Autodesk Fusion 360 part; units mm, degrees
note: some values were not read from the file. Set by a fixed rule: which sketch regions a step uses.
(part 7 of 8)
  spline S678 degree 3 poles (31.6566, -63.6923) (31.72, -63.6389) (31.7978, -63.6072) (31.8772, -63.5903) knots 0 0 0 0 1 1 1 1
  spline S679 degree 3 poles (31.8772, -63.5903) (31.9567, -63.5733) (32.0382, -63.5705) (32.1192, -63.568) knots 0 0 0 0 1 1 1 1
  line L146 (32.1192, -63.568) -> (36.4524, -63.4348)
  spline S680 degree 3 poles (36.4524, -63.4348) (36.4673, -62.5804) (36.8861, -61.7442) (37.5474, -61.2485) knots 0 0 0 0 1 1 1 1
  spline S681 degree 3 poles (37.5474, -61.2485) (37.8359, -61.0322) (38.1674, -60.8807) (38.5136, -60.8015) knots 0 0 0 0 1 1 1 1
  spline S682 degree 3 poles (38.5136, -60.8015) (38.8597, -60.7222) (39.217, -60.719) (39.5712, -60.7246) knots 0 0 0 0 1 1 1 1
  line L147 (39.5712, -60.7246) -> (51.3095, -60.9089)
  spline S683 degree 3 poles (51.3095, -60.9089) (51.8749, -60.9209) (52.434, -61.1493) (52.859, -61.542) knots 0 0 0 0 1 1 1 1
  spline S684 degree 3 poles (52.859, -61.542) (53.2166, -61.8724) (53.4741, -62.3063) (53.6869, -62.7542) knots 0 0 0 0 1 1 1 1
  spline S685 degree 3 poles (53.6869, -62.7542) (53.7992, -62.9906) (53.9007, -63.2329) (54.0258, -63.462) knots 0 0 0 0 1 1 1 1
  spline S686 degree 3 poles (54.0258, -63.462) (54.151, -63.691) (54.3018, -63.9085) (54.4972, -64.0744) knots 0 0 0 0 1 1 1 1
  spline S687 degree 3 poles (54.4972, -64.0744) (54.8359, -64.3623) (55.2785, -64.4726) (55.7089, -64.5418) knots 0 0 0 0 1 1 1 1
  spline S688 degree 3 poles (55.7089, -64.5418) (56.3802, -64.6497) (57.0608, -64.6746) (57.7397, -64.6945) knots 0 0 0 0 1 1 1 1
  line L148 (57.7397, -64.6945) -> (115.1827, -66.374)
  spline S689 degree 3 poles (115.1827, -66.374) (115.5699, -66.3854) (115.96, -66.4334) (116.3432, -66.374) knots 0 0 0 0 1 1 1 1
  spline S690 degree 3 poles (116.3432, -66.374) (116.6033, -66.3338) (116.8559, -66.2316) (117.0685, -66.0687) knots 0 0 0 0 1 1 1 1
  spline S691 degree 3 poles (117.0685, -66.0687) (117.4625, -65.7668) (117.6901, -65.2882) (117.9389, -64.8472) knots 0 0 0 0 1 1 1 1
  spline S692 degree 3 poles (117.9389, -64.8472) (118.221, -64.3467) (118.5582, -63.8627) (119.0216, -63.5455) knots 0 0 0 0 1 1 1 1
  spline S693 degree 3 poles (119.0216, -63.5455) (119.4371, -63.2611) (119.943, -63.126) (120.437, -63.1676) knots 0 0 0 0 1 1 1 1
  line L149 (120.437, -63.1676) -> (132.5399, -63.4822)
  spline S694 degree 3 poles (132.5399, -63.4822) (133.197, -63.4272) (133.8722, -63.6945) (134.3319, -64.1917) knots 0 0 0 0 1 1 1 1
  spline S695 degree 3 poles (134.3319, -64.1917) (134.8295, -64.7298) (135.0609, -65.5271) (134.934, -66.2661) knots 0 0 0 0 1 1 1 1
  line L150 (134.934, -66.2661) -> (139.3401, -66.482)
  spline S696 degree 3 poles (139.3401, -66.482) (139.4661, -66.4882) (139.593, -66.4946) (139.7157, -66.5251) knots 0 0 0 0 1 1 1 1
  spline S697 degree 3 poles (139.7157, -66.5251) (139.8385, -66.5557) (139.9582, -66.6121) (140.0478, -66.7056) knots 0 0 0 0 1 1 1 1
  spline S698 degree 3 poles (140.0478, -66.7056) (140.1454, -66.8077) (140.2011, -66.9477) (140.2275, -67.0899) knots 0 0 0 0 1 1 1 1
  spline S699 degree 3 poles (140.2275, -67.0899) (140.254, -67.2321) (140.2535, -67.3781) (140.2528, -67.5231) knots 0 0 0 0 1 1 1 1
  line L151 (140.2528, -67.5231) -> (140.2444, -69.6792)
  spline S700 degree 3 poles (140.2444, -69.6792) (140.2439, -69.7923) (140.2433, -69.906) (140.2607, -70.0175) knots 0 0 0 0 1 1 1 1
  spline S701 degree 3 poles (140.2607, -70.0175) (140.2782, -70.129) (140.3152, -70.2397) (140.3843, -70.3262) knots 0 0 0 0 1 1 1 1
  spline S702 degree 3 poles (140.3843, -70.3262) (140.4319, -70.3858) (140.4939, -70.4324) (140.5628, -70.4604) knots 0 0 0 0 1 1 1 1
  spline S703 degree 3 poles (140.5628, -70.4604) (140.6318, -70.4884) (140.7074, -70.4978) (140.7806, -70.4874) knots 0 0 0 0 1 1 1 1
  line L152 (140.7806, -70.4874) -> (144.4775, -70.5414)
  spline S704 degree 3 poles (144.4775, -70.5414) (144.6381, -70.5658) (144.8078, -70.5118) (144.9287, -70.398) knots 0 0 0 0 1 1 1 1
  spline S705 degree 3 poles (144.9287, -70.398) (145.0669, -70.2678) (145.1365, -70.0617) (145.1075, -69.869) knots 0 0 0 0 1 1 1 1
  line L153 (145.1075, -69.869) -> (145.2012, -67.102)
  spline S706 degree 3 poles (145.2012, -67.102) (145.388, -66.9765) (145.5898, -66.8756) (145.8003, -66.8025) knots 0 0 0 0 1 1 1 1
  spline S707 degree 3 poles (145.8003, -66.8025) (146.3846, -66.5995) (147.0308, -66.6173) (147.6149, -66.8209) knots 0 0 0 0 1 1 1 1
  spline S708 degree 3 poles (147.6149, -66.8209) (148.199, -67.0245) (148.7207, -67.4089) (149.1271, -67.8952) knots 0 0 0 0 1 1 1 1
  spline S709 degree 3 poles (149.1271, -67.8952) (149.9398, -68.8679) (150.2708, -70.2083) (150.2564, -71.5036) knots 0 0 0 0 1 1 1 1
  spline S710 degree 3 poles (150.2564, -71.5036) (150.2364, -73.3042) (149.5784, -75.0893) (148.4395, -76.433) knots 0 0 0 0 1 1 1 1
  line L154 (148.4395, -76.433) -> (134.4244, -76.4161)
  spline S711 degree 3 poles (134.4244, -76.4161) (134.2986, -76.8823) (133.9928, -77.2916) (133.5922, -77.5304) knots 0 0 0 0 1 1 1 1
  spline S712 degree 3 poles (133.5922, -77.5304) (133.3009, -77.704) (132.9679, -77.7878) (132.6349, -77.8227) knots 0 0 0 0 1 1 1 1
  spline S713 degree 3 poles (132.6349, -77.8227) (132.3018, -77.8576) (131.9661, -77.846) (131.6316, -77.835) knots 0 0 0 0 1 1 1 1
  line L155 (131.6316, -77.835) -> (116.301, -77.3322)
  spline S714 degree 3 poles (116.301, -77.3322) (116.0942, -77.3254) (115.8862, -77.3195) (115.6817, -77.352) knots 0 0 0 0 1 1 1 1
  spline S715 degree 3 poles (115.6817, -77.352) (115.4771, -77.3844) (115.275, -77.4566) (115.1097, -77.5874) knots 0 0 0 0 1 1 1 1
  spline S716 degree 3 poles (115.1097, -77.5874) (114.9652, -77.7018) (114.8519, -77.8595) (114.7868, -78.0371) knots 0 0 0 0 1 1 1 1
  spline S717 degree 3 poles (114.7868, -78.0371) (114.7217, -78.2146) (114.7049, -78.4115) (114.7391, -78.5984) knots 0 0 0 0 1 1 1 1
  line L156 (114.7391, -78.5984) -> (114.679, -87.6426)
  spline S718 degree 3 poles (114.679, -87.6426) (114.6256, -88.1512) (114.8192, -88.6818) (115.1823, -89.0222) knots 0 0 0 0 1 1 1 1
  spline S719 degree 3 poles (115.1823, -89.0222) (115.4591, -89.2817) (115.8278, -89.4297) (116.1985, -89.4301) knots 0 0 0 0 1 1 1 1
  line L157 (116.1985, -89.4301) -> (132.3849, -90.0671)
  spline S720 degree 3 poles (132.3849, -90.0671) (132.8554, -90.0523) (133.3293, -90.2173) (133.6985, -90.5247) knots 0 0 0 0 1 1 1 1
  spline S721 degree 3 poles (133.6985, -90.5247) (134.111, -90.8681) (134.3875, -91.3869) (134.4509, -91.9364) knots 0 0 0 0 1 1 1 1
  line L158 (134.4509, -91.9364) -> (148.0775, -92.4299)
  spline S722 degree 3 poles (148.0775, -92.4299) (148.7841, -93.2593) (149.2811, -94.2848) (149.5041, -95.3738) knots 0 0 0 0 1 1 1 1
  spline S723 degree 3 poles (149.5041, -95.3738) (149.7272, -96.4628) (149.6758, -97.6127) (149.3567, -98.6748) knots 0 0 0 0 1 1 1 1
  spline S724 degree 3 poles (149.3567, -98.6748) (149.037, -99.7388) (148.4265, -100.7358) (147.5295, -101.3306) knots 0 0 0 0 1 1 1 1
  spline S725 degree 3 poles (147.5295, -101.3306) (146.6734, -101.8983) (145.5839, -102.0595) (144.6123, -101.7625) knots 0 0 0 0 1 1 1 1
  line L159 (144.6123, -101.7625) -> (144.4848, -98.6994)
  spline S726 degree 3 poles (144.4848, -98.6994) (144.4471, -98.4963) (144.3395, -98.3083) (144.1866, -98.1781) knots 0 0 0 0 1 1 1 1
  spline S727 degree 3 poles (144.1866, -98.1781) (144.045, -98.0575) (143.8654, -97.9871) (143.6833, -97.9807) knots 0 0 0 0 1 1 1 1
  line L160 (143.6833, -97.9807) -> (139.8253, -98.044)
  spline S728 degree 3 poles (139.8253, -98.044) (139.7385, -98.0222) (139.645, -98.0305) (139.5628, -98.0672) knots 0 0 0 0 1 1 1 1
  spline S729 degree 3 poles (139.5628, -98.0672) (139.4806, -98.1039) (139.41, -98.1689) (139.3645, -98.2498) knots 0 0 0 0 1 1 1 1
  spline S730 degree 3 poles (139.3645, -98.2498) (139.312, -98.3432) (139.2936, -98.4573) (139.314, -98.5637) knots 0 0 0 0 1 1 1 1
  line L161 (139.314, -98.5637) -> (139.2927, -101.0538)
  spline S731 degree 3 poles (139.2927, -101.0538) (139.2918, -101.1632) (139.2919, -101.2731) (139.2754, -101.3811) knots 0 0 0 0 1 1 1 1
  spline S732 degree 3 poles (139.2754, -101.3811) (139.259, -101.4891) (139.2237, -101.5973) (139.1538, -101.6781) knots 0 0 0 0 1 1 1 1
  spline S733 degree 3 poles (139.1538, -101.6781) (139.099, -101.7413) (139.0241, -101.7849) (138.9441, -101.8) knots 0 0 0 0 1 1 1 1
  spline S734 degree 3 poles (138.9441, -101.8) (138.8641, -101.8151) (138.7795, -101.8018) (138.7072, -101.7625) knots 0 0 0 0 1 1 1 1
  line L162 (138.7072, -101.7625) -> (134.1943, -101.727)
  spline S735 degree 3 poles (134.1943, -101.727) (134.229, -102.4331) (133.9527, -103.1494) (133.4602, -103.6302) knots 0 0 0 0 1 1 1 1
  spline S736 degree 3 poles (133.4602, -103.6302) (132.9548, -104.1237) (132.2312, -104.3585) (131.5496, -104.2503) knots 0 0 0 0 1 1 1 1
  line L163 (131.5496, -104.2503) -> (119.2196, -103.9449)
  spline S737 degree 3 poles (119.2196, -103.9449) (118.7058, -103.8469) (118.2103, -103.6435) (117.7691, -103.3496) knots 0 0 0 0 1 1 1 1
  spline S738 degree 3 poles (117.7691, -103.3496) (116.7604, -102.6777) (116.059, -101.5174) (115.9082, -100.2711) knots 0 0 0 0 1 1 1 1
  line L164 (115.9082, -100.2711) -> (56.2497, -98.6007)
  spline S739 degree 3 poles (56.2497, -98.6007) (55.8137, -98.5885) (55.3761, -98.5631) (54.9424, -98.6108) knots 0 0 0 0 1 1 1 1
  spline S740 degree 3 poles (54.9424, -98.6108) (54.6257, -98.6457) (54.3104, -98.7254) (54.0276, -98.8796) knots 0 0 0 0 1 1 1 1
  spline S741 degree 3 poles (54.0276, -98.8796) (53.7288, -99.0426) (53.4681, -99.292) (53.3121, -99.6058) knots 0 0 0 0 1 1 1 1
  spline S742 degree 3 poles (53.3121, -99.6058) (53.1309, -99.9701) (53.0969, -100.4001) (52.9144, -100.7635) knots 0 0 0 0 1 1 1 1
  spline S743 degree 3 poles (52.9144, -100.7635) (52.7902, -101.0109) (52.5983, -101.2201) (52.3677, -101.3593) knots 0 0 0 0 1 1 1 1
  spline S744 degree 3 poles (52.3677, -101.3593) (52.1372, -101.4986) (51.8688, -101.5676) (51.6033, -101.5558) knots 0 0 0 0 1 1 1 1
  line L165 (51.6033, -101.5558) -> (38.2697, -101.3753)
  spline S745 degree 3 poles (38.2697, -101.3753) (38.091, -101.3728) (37.9112, -101.3654) (37.7366, -101.3251) knots 0 0 0 0 1 1 1 1
  spline S746 degree 3 poles (37.7366, -101.3251) (37.5619, -101.2848) (37.3942, -101.2146) (37.2367, -101.1255) knots 0 0 0 0 1 1 1 1
  spline S747 degree 3 poles (37.2367, -101.1255) (36.7988, -100.8776) (36.4344, -100.4879) (36.2061, -100.023) knots 0 0 0 0 1 1 1 1
  spline S748 degree 3 poles (36.2061, -100.023) (35.9777, -99.558) (35.8862, -99.0198) (35.9473, -98.5004) knots 0 0 0 0 1 1 1 1
  line L166 (35.9473, -98.5004) -> (31.6028, -98.5729)
  spline S749 degree 3 poles (31.6028, -98.5729) (31.5017, -98.5746) (31.4001, -98.5759) (31.2999, -98.5609) knots 0 0 0 0 1 1 1 1
  spline S750 degree 3 poles (31.2999, -98.5609) (31.1998, -98.5459) (31.1007, -98.5143) (31.0153, -98.4572) knots 0 0 0 0 1 1 1 1
  spline S751 degree 3 poles (31.0153, -98.4572) (30.9306, -98.4006) (30.8609, -98.3193) (30.816, -98.2248) knots 0 0 0 0 1 1 1 1
  spline S752 degree 3 poles (30.816, -98.2248) (30.7711, -98.1302) (30.7511, -98.0228) (30.7589, -97.9174) knots 0 0 0 0 1 1 1 1
  line L167 (30.7589, -97.9174) -> (30.5626, -95.1243)
  spline S753 degree 3 poles (30.5626, -95.1243) (30.5691, -94.9213) (30.497, -94.7167) (30.3662, -94.5675) knots 0 0 0 0 1 1 1 1
  spline S754 degree 3 poles (30.3662, -94.5675) (30.2314, -94.4137) (30.036, -94.3208) (29.8373, -94.3161) knots 0 0 0 0 1 1 1 1
  line L168 (29.8373, -94.3161) -> (26.5346, -94.3161)
  spline S755 degree 3 poles (26.5346, -94.3161) (26.345, -94.3013) (26.1506, -94.3833) (26.0233, -94.532) knots 0 0 0 0 1 1 1 1
  spline S756 degree 3 poles (26.0233, -94.532) (25.8998, -94.6763) (25.8418, -94.88) (25.8694, -95.0719) knots 0 0 0 0 1 1 1 1
  line L169 (25.8694, -95.0719) -> (25.8958, -98.1781)
  spline S757 degree 3 poles (25.8958, -98.1781) (25.7078, -98.2397) (25.5151, -98.2852) (25.3201, -98.3138) knots 0 0 0 0 1 1 1 1
  spline S758 degree 3 poles (25.3201, -98.3138) (24.1359, -98.4877) (22.9011, -98.0083) (22.0407, -97.1343) knots 0 0 0 0 1 1 1 1
  spline S759 degree 3 poles (22.0407, -97.1343) (21.1803, -96.2604) (20.6873, -95.0226) (20.6018, -93.7673) knots 0 0 0 0 1 1 1 1
  spline S760 degree 3 poles (20.6018, -93.7673) (20.5342, -92.7749) (20.7118, -91.7652) (21.1125, -90.8641) knots 0 0 0 0 1 1 1 1
  spline S761 degree 3 poles (21.1125, -90.8641) (21.5132, -89.9631) (22.136, -89.1727) (22.9032, -88.5916) knots 0 0 0 0 1 1 1 1
  line L170 (22.9032, -88.5916) -> (36.0426, -88.6126)
  spline S762 degree 3 poles (36.0426, -88.6126) (36.2305, -88.291) (36.4815, -88.0104) (36.7752, -87.7936) knots 0 0 0 0 1 1 1 1
  spline S763 degree 3 poles (36.7752, -87.7936) (37.301, -87.4054) (37.9646, -87.2295) (38.6024, -87.3093) knots 0 0 0 0 1 1 1 1
  line L171 (38.6024, -87.3093) -> (54.207, -87.5792)
  spline S764 degree 3 poles (54.207, -87.5792) (54.4119, -87.5828) (54.6169, -87.5896) (54.8215, -87.5788) knots 0 0 0 0 1 1 1 1
  spline S765 degree 3 poles (54.8215, -87.5788) (55.0261, -87.568) (55.2334, -87.5368) (55.4188, -87.445) knots 0 0 0 0 1 1 1 1
  spline S766 degree 3 poles (55.4188, -87.445) (55.5846, -87.363) (55.7285, -87.2325) (55.8301, -87.0721) knots 0 0 0 0 1 1 1 1
  spline S767 degree 3 poles (55.8301, -87.0721) (55.9318, -86.9116) (55.9909, -86.7216) (55.999, -86.5289) knots 0 0 0 0 1 1 1 1
  line L172 (55.999, -86.5289) -> (56.084, -76.945)
  spline S768 degree 3 poles (56.084, -76.945) (56.1246, -76.6242) (56.04, -76.288) (55.854, -76.0304) knots 0 0 0 0 1 1 1 1
  spline S769 degree 3 poles (55.854, -76.0304) (55.7351, -75.8658) (55.5764, -75.7333) (55.3971, -75.6489) knots 0 0 0 0 1 1 1 1
  spline S770 degree 3 poles (55.3971, -75.6489) (55.2178, -75.5644) (55.0183, -75.5282) (54.8225, -75.5446) knots 0 0 0 0 1 1 1 1
  line L173 (54.8225, -75.5446) -> (39.1987, -75.0866)
  spline S771 degree 3 poles (39.1987, -75.0866) (38.6749, -75.0881) (38.1519, -74.9167) (37.7217, -74.6023) knots 0 0 0 0 1 1 1 1
  spline S772 degree 3 poles (37.7217, -74.6023) (37.2306, -74.2434) (36.8646, -73.6992) (36.7063, -73.0923) knots 0 0 0 0 1 1 1 1
  line L174 (36.7063, -73.0923) -> (23.3609, -72.9778)
  spline S773 degree 3 poles (61.6096, -85.4144) (62.5092, -85.697) (63.5138, -85.5881) (64.3398, -85.1184) knots 0 0 0 0 1 1 1 1
  spline S774 degree 3 poles (64.3398, -85.1184) (65.1657, -84.6487) (65.803, -83.824) (66.0715, -82.8771) knots 0 0 0 0 1 1 1 1
  spline S775 degree 3 poles (66.0715, -82.8771) (66.34, -81.9302) (66.2366, -80.8728) (65.7903, -80.0033) knots 0 0 0 0 1 1 1 1
  spline S776 degree 3 poles (65.7903, -80.0033) (65.3441, -79.1339) (64.5606, -78.4632) (63.6611, -78.1805) knots 0 0 0 0 1 1 1 1
  spline S777 degree 3 poles (63.6611, -78.1805) (62.7615, -77.8979) (61.7569, -78.0068) (60.9309, -78.4764) knots 0 0 0 0 1 1 1 1
  spline S778 degree 3 poles (60.9309, -78.4764) (60.1049, -78.9461) (59.4677, -79.7709) (59.1992, -80.7178) knots 0 0 0 0 1 1 1 1
  spline S779 degree 3 poles (59.1992, -80.7178) (58.9307, -81.6647) (59.0341, -82.7221) (59.4803, -83.5915) knots 0 0 0 0 1 1 1 1
  spline S780 degree 3 poles (59.4803, -83.5915) (59.9265, -84.461) (60.71, -85.1317) (61.6096, -85.4144) knots 0 0 0 0 1 1 1 1
  spline S781 degree 3 poles (107.0492, -86.9394) (107.9487, -87.2221) (108.9533, -87.1132) (109.7793, -86.6435) knots 0 0 0 0 1 1 1 1
  spline S782 degree 3 poles (109.7793, -86.6435) (110.6053, -86.1738) (111.2425, -85.3491) (111.511, -84.4022) knots 0 0 0 0 1 1 1 1
  spline S783 degree 3 poles (111.511, -84.4022) (111.7796, -83.4553) (111.6761, -82.3979) (111.2299, -81.5284) knots 0 0 0 0 1 1 1 1
  spline S784 degree 3 poles (111.2299, -81.5284) (110.7837, -80.659) (110.0002, -79.9883) (109.1006, -79.7056) knots 0 0 0 0 1 1 1 1
  spline S785 degree 3 poles (109.1006, -79.7056) (108.201, -79.4229) (107.1964, -79.5318) (106.3704, -80.0015) knots 0 0 0 0 1 1 1 1
  spline S786 degree 3 poles (106.3704, -80.0015) (105.5445, -80.4712) (104.9073, -81.2959) (104.6387, -82.2428) knots 0 0 0 0 1 1 1 1
  spline S787 degree 3 poles (104.6387, -82.2428) (104.3702, -83.1898) (104.4737, -84.2472) (104.9199, -85.1166) knots 0 0 0 0 1 1 1 1
  spline S788 degree 3 poles (104.9199, -85.1166) (105.3661, -85.9861) (106.1496, -86.6568) (107.0492, -86.9394) knots 0 0 0 0 1 1 1 1
  spline S789 degree 3 poles (70.4142, -72.9585) (70.125, -72.9646) (69.8399, -73.0954) (69.6387, -73.3143) knots 0 0 0 0 1 1 1 1
  spline S790 degree 3 poles (69.6387, -73.3143) (69.4375, -73.5331) (69.3226, -73.8373) (69.3263, -74.1418) knots 0 0 0 0 1 1 1 1
  spline S791 degree 3 poles (69.3263, -74.1418) (69.3292, -74.3898) (69.4096, -74.6361) (69.5519, -74.8336) knots 0 0 0 0 1 1 1 1
  spline S792 degree 3 poles (69.5519, -74.8336) (69.6943, -75.0312) (69.898, -75.179) (70.1241, -75.2488) knots 0 0 0 0 1 1 1 1
  line L175 (70.1241, -75.2488) -> (100.8764, -75.8977)
  spline S793 degree 3 poles (100.8764, -75.8977) (101.0768, -75.8592) (101.2658, -75.7576) (101.413, -75.6094) knots 0 0 0 0 1 1 1 1
  spline S794 degree 3 poles (101.413, -75.6094) (101.5602, -75.4612) (101.665, -75.2669) (101.7105, -75.058) knots 0 0 0 0 1 1 1 1
  spline S795 degree 3 poles (101.7105, -75.058) (101.7872, -74.7058) (101.6866, -74.3163) (101.4511, -74.0535) knots 0 0 0 0 1 1 1 1
  spline S796 degree 3 poles (101.4511, -74.0535) (101.2157, -73.7906) (100.8522, -73.662) (100.5137, -73.7219) knots 0 0 0 0 1 1 1 1
  line L176 (100.5137, -73.7219) -> (99.6071, -73.6837)
  line L177 (99.6071, -73.6837) -> (99.6434, -74.1036)
  line L178 (99.6434, -74.1036) -> (97.6488, -74.1036)
  line L179 (97.6488, -74.1036) -> (97.6488, -73.6456)
  line L180 (97.6488, -73.6456) -> (95.9807, -73.6074)
  line L181 (95.9807, -73.6074) -> (95.9807, -74.0655)
  line L182 (95.9807, -74.0655) -> (93.8411, -74.0655)
  line L183 (93.8411, -74.0655) -> (93.8048, -73.5311)
  line L184 (93.8048, -73.5311) -> (92.2092, -73.5311)
  line L185 (92.2092, -73.5311) -> (92.2092, -74.0273)
  line L186 (92.2092, -74.0273) -> (90.1058, -73.9509)
  line L187 (90.1058, -73.9509) -> (90.1421, -73.4547)
  line L188 (90.1421, -73.4547) -> (88.5827, -73.3784)
  line L189 (88.5827, -73.3784) -> (88.5827, -73.8364)
  line L190 (88.5827, -73.8364) -> (86.5156, -73.7601)
  line L191 (86.5156, -73.7601) -> (86.5156, -73.3402)
  line L192 (86.5156, -73.3402) -> (84.7749, -73.3402)
  line L193 (84.7749, -73.3402) -> (84.8112, -73.7219)
  line L194 (84.8112, -73.7219) -> (82.6716, -73.6074)
  line L195 (82.6716, -73.6074) -> (82.6716, -73.1494)
  line L196 (82.6716, -73.1494) -> (81.0034, -73.1112)
  line L197 (81.0034, -73.1112) -> (81.0034, -73.6074)
  line L198 (81.0034, -73.6074) -> (78.9726, -73.5692)
  line L199 (78.9726, -73.5692) -> (79.0089, -73.1112)
  line L200 (79.0089, -73.1112) -> (77.0869, -73.1112)
  line L201 (77.0869, -73.1112) -> (77.1231, -73.5311)
  line L202 (77.1231, -73.5311) -> (75.1648, -73.4547)
  line L203 (75.1648, -73.4547) -> (75.1648, -72.9966)
  line L204 (75.1648, -72.9966) -> (73.3516, -72.9585)
  line L205 (73.3516, -72.9585) -> (73.3516, -73.4165)
  line L206 (73.3516, -73.4165) -> (71.4296, -73.3784)
  line L207 (71.4296, -73.3784) -> (71.4659, -72.9585)
  line L208 (71.4659, -72.9585) -> (70.4142, -72.9585)
  spline S797 degree 3 poles (70.1838, -88.8776) (69.8946, -88.8838) (69.6095, -89.0146) (69.4083, -89.2334) knots 0 0 0 0 1 1 1 1
  spline S798 degree 3 poles (69.4083, -89.2334) (69.2071, -89.4522) (69.0922, -89.7565) (69.0959, -90.061) knots 0 0 0 0 1 1 1 1
  spline S799 degree 3 poles (69.0959, -90.061) (69.0988, -90.3089) (69.1792, -90.5552) (69.3216, -90.7528) knots 0 0 0 0 1 1 1 1
  spline S800 degree 3 poles (69.3216, -90.7528) (69.4639, -90.9504) (69.6676, -91.0982) (69.8937, -91.168) knots 0 0 0 0 1 1 1 1
  line L209 (69.8937, -91.168) -> (100.646, -91.8169)
  spline S801 degree 3 poles (100.646, -91.8169) (100.8464, -91.7783) (101.0354, -91.6767) (101.1826, -91.5285) knots 0 0 0 0 1 1 1 1
  spline S802 degree 3 poles (101.1826, -91.5285) (101.3298, -91.3804) (101.4346, -91.1861) (101.4801, -90.9771) knots 0 0 0 0 1 1 1 1
  spline S803 degree 3 poles (101.4801, -90.9771) (101.5568, -90.6249) (101.4562, -90.2355) (101.2208, -89.9726) knots 0 0 0 0 1 1 1 1
  spline S804 degree 3 poles (101.2208, -89.9726) (100.9853, -89.7097) (100.6219, -89.5812) (100.2834, -89.6411) knots 0 0 0 0 1 1 1 1
  line L210 (100.2834, -89.6411) -> (99.3767, -89.6029)
  line L211 (99.3767, -89.6029) -> (99.413, -90.0228)
  line L212 (99.413, -90.0228) -> (97.4185, -90.0228)
  line L213 (97.4185, -90.0228) -> (97.4185, -89.5647)
  line L214 (97.4185, -89.5647) -> (95.7503, -89.5265)
  line L215 (95.7503, -89.5265) -> (95.7503, -89.9846)
  line L216 (95.7503, -89.9846) -> (93.6107, -89.9846)
  line L217 (93.6107, -89.9846) -> (93.5744, -89.4502)
  line L218 (93.5744, -89.4502) -> (91.9788, -89.4502)
  line L219 (91.9788, -89.4502) -> (91.9788, -89.9464)
  line L220 (91.9788, -89.9464) -> (89.8754, -89.8701)
  line L221 (89.8754, -89.8701) -> (89.9117, -89.3738)
  line L222 (89.9117, -89.3738) -> (88.3523, -89.2975)
  line L223 (88.3523, -89.2975) -> (88.3523, -89.7556)
  line L224 (88.3523, -89.7556) -> (86.2852, -89.6792)
  line L225 (86.2852, -89.6792) -> (86.2853, -89.2593)
  line L226 (86.2853, -89.2593) -> (84.5445, -89.2593)
  line L227 (84.5445, -89.2593) -> (84.5808, -89.6411)
  line L228 (84.5808, -89.6411) -> (82.4412, -89.5266)
  line L229 (82.4412, -89.5266) -> (82.4412, -89.0685)
  line L230 (82.4412, -89.0685) -> (80.773, -89.0303)
  line L231 (80.773, -89.0303) -> (80.773, -89.5266)
  line L232 (80.773, -89.5266) -> (78.7422, -89.4884)
  line L233 (78.7422, -89.4884) -> (78.7785, -89.0303)
  line L234 (78.7785, -89.0303) -> (76.8565, -89.0303)
  line L235 (76.8565, -89.0303) -> (76.8927, -89.4502)
  line L236 (76.8927, -89.4502) -> (74.9345, -89.3739)
  line L237 (74.9345, -89.3739) -> (74.9345, -88.9158)
  line L238 (74.9345, -88.9158) -> (73.1212, -88.8776)
  line L239 (73.1212, -88.8776) -> (73.1212, -89.3357)
  line L240 (73.1212, -89.3357) -> (71.1992, -89.2975)
  line L241 (71.1992, -89.2975) -> (71.2355, -88.8776)
  line L242 (71.2355, -88.8776) -> (70.1838, -88.8776)
  spline S805 degree 3 poles (40.0385, -65.8564) (39.8943, -65.8457) (39.747, -65.8893) (39.6293, -65.9775) knots 0 0 0 0 1 1 1 1
  spline S806 degree 3 poles (39.6293, -65.9775) (39.4979, -66.0759) (39.4048, -66.2294) (39.3754, -66.3962) knots 0 0 0 0 1 1 1 1
  line L243 (39.3754, -66.3962) -> (39.3516, -69.1652)
  spline S807 degree 3 poles (39.3516, -69.1652) (39.3441, -69.3712) (39.4172, -69.5791) (39.5505, -69.7301) knots 0 0 0 0 1 1 1 1
  spline S808 degree 3 poles (39.5505, -69.7301) (39.7053, -69.9056) (39.9394, -69.9997) (40.1659, -69.9777) knots 0 0 0 0 1 1 1 1
  line L244 (40.1659, -69.9777) -> (49.2948, -69.9461)
  spline S809 degree 3 poles (49.2948, -69.9461) (49.7336, -69.8277) (50.1315, -69.5479) (50.4034, -69.1665) knots 0 0 0 0 1 1 1 1
  spline S810 degree 3 poles (50.4034, -69.1665) (50.6752, -68.7851) (50.8192, -68.3047) (50.8044, -67.8281) knots 0 0 0 0 1 1 1 1
  spline S811 degree 3 poles (50.8044, -67.8281) (50.7896, -67.3516) (50.6163, -66.8822) (50.3215, -66.5203) knots 0 0 0 0 1 1 1 1
  spline S812 degree 3 poles (50.3215, -66.5203) (50.0267, -66.1583) (49.6125, -65.9064) (49.1673, -65.8183) knots 0 0 0 0 1 1 1 1
  line L245 (49.1673, -65.8183) -> (40.0385, -65.8564)
  spline S813 degree 3 poles (39.4634, -92.3493) (39.3192, -92.3386) (39.1719, -92.3822) (39.0542, -92.4704) knots 0 0 0 0 1 1 1 1
  spline S814 degree 3 poles (39.0542, -92.4704) (38.9228, -92.5688) (38.8298, -92.7223) (38.8003, -92.8892) knots 0 0 0 0 1 1 1 1
  line L246 (38.8003, -92.8892) -> (38.7765, -95.6581)
  spline S815 degree 3 poles (38.7765, -95.6581) (38.769, -95.8641) (38.8422, -96.0721) (38.9754, -96.2231) knots 0 0 0 0 1 1 1 1
  spline S816 degree 3 poles (38.9754, -96.2231) (39.1302, -96.3985) (39.3644, -96.4927) (39.5908, -96.4706) knots 0 0 0 0 1 1 1 1
  line L247 (39.5908, -96.4706) -> (48.7197, -96.439)
  spline S817 degree 3 poles (48.7197, -96.439) (49.1585, -96.3206) (49.5564, -96.0408) (49.8283, -95.6594) knots 0 0 0 0 1 1 1 1
  spline S818 degree 3 poles (49.8283, -95.6594) (50.1002, -95.278) (50.2441, -94.7976) (50.2293, -94.321) knots 0 0 0 0 1 1 1 1
  spline S819 degree 3 poles (50.2293, -94.321) (50.2146, -93.8445) (50.0412, -93.3751) (49.7464, -93.0132) knots 0 0 0 0 1 1 1 1
  spline S820 degree 3 poles (49.7464, -93.0132) (49.4516, -92.6513) (49.0374, -92.3993) (48.5923, -92.3112) knots 0 0 0 0 1 1 1 1
  line L248 (48.5923, -92.3112) -> (39.4634, -92.3493)
  spline S821 degree 3 poles (120.9015, -94.8805) (120.7574, -94.868) (120.6097, -94.9097) (120.4909, -94.9964) knots 0 0 0 0 1 1 1 1
  spline S822 degree 3 poles (120.4909, -94.9964) (120.3584, -95.0931) (120.2636, -95.2454) (120.2323, -95.4119) knots 0 0 0 0 1 1 1 1
  line L249 (120.2323, -95.4119) -> (120.1767, -98.1804)
  spline S823 degree 3 poles (120.1767, -98.1804) (120.1671, -98.3862) (120.2376, -98.5951) (120.3691, -98.7478) knots 0 0 0 0 1 1 1 1
  spline S824 degree 3 poles (120.3691, -98.7478) (120.5219, -98.9252) (120.7549, -99.0223) (120.9816, -99.0031) knots 0 0 0 0 1 1 1 1
  line L250 (120.9816, -99.0031) -> (130.1102, -99.0875)
  spline S825 degree 3 poles (130.1102, -99.0875) (130.5504, -98.9747) (130.9514, -98.6999) (131.2276, -98.322) knots 0 0 0 0 1 1 1 1
  spline S826 degree 3 poles (131.2276, -98.322) (131.5038, -97.944) (131.6533, -97.4655) (131.644, -96.9888) knots 0 0 0 0 1 1 1 1
  spline S827 degree 3 poles (131.644, -96.9888) (131.6344, -96.5121) (131.4667, -96.0406) (131.1761, -95.6749) knots 0 0 0 0 1 1 1 1
  spline S828 degree 3 poles (131.1761, -95.6749) (130.8855, -95.3093) (130.4741, -95.0521) (130.0301, -94.9583) knots 0 0 0 0 1 1 1 1
  line L251 (130.0301, -94.9583) -> (120.9015, -94.8805)
  spline S829 degree 3 poles (121.5447, -68.1469) (121.3998, -68.1377) (121.2523, -68.1827) (121.1346, -68.272) knots 0 0 0 0 1 1 1 1
  spline S830 degree 3 poles (121.1346, -68.272) (120.9978, -68.3759) (120.903, -68.5392) (120.8778, -68.7147) knots 0 0 0 0 1 1 1 1
  line L252 (120.8778, -68.7147) -> (120.8343, -71.6554)
  spline S831 degree 3 poles (120.8343, -71.6554) (120.819, -71.8725) (120.8911, -72.095) (121.0293, -72.2571) knots 0 0 0 0 1 1 1 1
  spline S832 degree 3 poles (121.0293, -72.2571) (121.1822, -72.4364) (121.4143, -72.5378) (121.6429, -72.5251) knots 0 0 0 0 1 1 1 1
  line L253 (121.6429, -72.5251) -> (130.7718, -72.5676)
  spline S833 degree 3 poles (130.7718, -72.5676) (131.2188, -72.4219) (131.6182, -72.119) (131.891, -71.7187) knots 0 0 0 0 1 1 1 1
  spline S834 degree 3 poles (131.891, -71.7187) (132.1638, -71.3185) (132.3084, -70.8232) (132.2963, -70.3307) knots 0 0 0 0 1 1 1 1
  spline S835 degree 3 poles (132.2963, -70.3307) (132.2843, -69.84) (132.1167, -69.355) (131.8264, -68.9708) knots 0 0 0 0 1 1 1 1
  spline S836 degree 3 poles (131.8264, -68.9708) (131.5362, -68.5866) (131.125, -68.3054) (130.6735, -68.1825) knots 0 0 0 0 1 1 1 1
  line L254 (130.6735, -68.1825) -> (121.5447, -68.1469)
  spline S837 degree 3 poles (50.922, -73.3977) (50.7287, -73.343) (50.5131, -73.371) (50.3444, -73.4845) knots 0 0 0 0 1 1 1 1
  spline S838 degree 3 poles (50.3444, -73.4845) (50.2601, -73.5412) (50.188, -73.6183) (50.1368, -73.7088) knots 0 0 0 0 1 1 1 1
  spline S839 degree 3 poles (50.1368, -73.7088) (50.0856, -73.7993) (50.0555, -73.9032) (50.0516, -74.0085) knots 0 0 0 0 1 1 1 1
  spline S840 degree 3 poles (50.0516, -74.0085) (50.0478, -74.1116) (50.0692, -74.2154) (50.1118, -74.3084) knots 0 0 0 0 1 1 1 1
  spline S841 degree 3 poles (50.1118, -74.3084) (50.1543, -74.4013) (50.2179, -74.4833) (50.295, -74.5471) knots 0 0 0 0 1 1 1 1
  spline S842 degree 3 poles (50.295, -74.5471) (50.4491, -74.6746) (50.6555, -74.7256) (50.8495, -74.6956) knots 0 0 0 0 1 1 1 1
  spline S843 degree 3 poles (50.8495, -74.6956) (50.9958, -74.673) (51.1367, -74.6051) (51.2432, -74.497) knots 0 0 0 0 1 1 1 1
  spline S844 degree 3 poles (51.2432, -74.497) (51.3496, -74.3889) (51.4199, -74.2402) (51.4297, -74.0848) knots 0 0 0 0 1 1 1 1
  spline S845 degree 3 poles (51.4297, -74.0848) (51.4395, -73.928) (51.3873, -73.7693) (51.2935, -73.647) knots 0 0 0 0 1 1 1 1
  spline S846 degree 3 poles (51.2935, -73.647) (51.1997, -73.5247) (51.0662, -73.4386) (50.922, -73.3977) knots 0 0 0 0 1 1 1 1
  spline S847 degree 3 poles (50.6677, -88.1798) (50.4744, -88.1251) (50.2589, -88.1531) (50.0902, -88.2666) knots 0 0 0 0 1 1 1 1
  spline S848 degree 3 poles (50.0902, -88.2666) (50.0059, -88.3233) (49.9337, -88.4004) (49.8825, -88.4909) knots 0 0 0 0 1 1 1 1
  spline S849 degree 3 poles (49.8825, -88.4909) (49.8313, -88.5814) (49.8013, -88.6853) (49.7974, -88.7906) knots 0 0 0 0 1 1 1 1
  spline S850 degree 3 poles (49.7974, -88.7906) (49.7936, -88.8937) (49.815, -88.9975) (49.8575, -89.0905) knots 0 0 0 0 1 1 1 1
  spline S851 degree 3 poles (49.8575, -89.0905) (49.9001, -89.1834) (49.9637, -89.2654) (50.0408, -89.3292) knots 0 0 0 0 1 1 1 1
  spline S852 degree 3 poles (50.0408, -89.3292) (50.1949, -89.4567) (50.4012, -89.5077) (50.5952, -89.4777) knots 0 0 0 0 1 1 1 1
  spline S853 degree 3 poles (50.5952, -89.4777) (50.7415, -89.4551) (50.8825, -89.3872) (50.9889, -89.2791) knots 0 0 0 0 1 1 1 1
  spline S854 degree 3 poles (50.9889, -89.2791) (51.0954, -89.171) (51.1657, -89.0223) (51.1754, -88.8669) knots 0 0 0 0 1 1 1 1
  spline S855 degree 3 poles (51.1754, -88.8669) (51.1853, -88.7101) (51.1331, -88.5514) (51.0393, -88.4291) knots 0 0 0 0 1 1 1 1
  spline S856 degree 3 poles (51.0393, -88.4291) (50.9455, -88.3068) (50.8119, -88.2207) (50.6677, -88.1798) knots 0 0 0 0 1 1 1 1
  spline S857 degree 3 poles (120.0781, -75.6593) (119.8848, -75.6046) (119.6692, -75.6326) (119.5005, -75.746) knots 0 0 0 0 1 1 1 1
  spline S858 degree 3 poles (119.5005, -75.746) (119.4162, -75.8028) (119.3441, -75.8799) (119.2929, -75.9704) knots 0 0 0 0 1 1 1 1
  spline S859 degree 3 poles (119.2929, -75.9704) (119.2417, -76.0609) (119.2116, -76.1648) (119.2077, -76.2701) knots 0 0 0 0 1 1 1 1
  spline S860 degree 3 poles (119.2077, -76.2701) (119.2035, -76.3732) (119.2253, -76.477) (119.2679, -76.57) knots 0 0 0 0 1 1 1 1
  spline S861 degree 3 poles (119.2679, -76.57) (119.3104, -76.6629) (119.374, -76.7449) (119.4511, -76.8087) knots 0 0 0 0 1 1 1 1
  spline S862 degree 3 poles (119.4511, -76.8087) (119.6052, -76.9362) (119.8116, -76.9872) (120.0055, -76.9572) knots 0 0 0 0 1 1 1 1
  spline S863 degree 3 poles (120.0055, -76.9572) (120.1519, -76.9345) (120.2928, -76.8667) (120.3993, -76.7586) knots 0 0 0 0 1 1 1 1
  spline S864 degree 3 poles (120.3993, -76.7586) (120.5057, -76.6505) (120.576, -76.5018) (120.5858, -76.3464) knots 0 0 0 0 1 1 1 1
  spline S865 degree 3 poles (120.5858, -76.3464) (120.5953, -76.1896) (120.5434, -76.0309) (120.4496, -75.9086) knots 0 0 0 0 1 1 1 1
  spline S866 degree 3 poles (120.4496, -75.9086) (120.3559, -75.7863) (120.2223, -75.7002) (120.0781, -75.6593) knots 0 0 0 0 1 1 1 1
  spline S867 degree 3 poles (119.7154, -90.3175) (119.5221, -90.2627) (119.3066, -90.2908) (119.1379, -90.4042) knots 0 0 0 0 1 1 1 1
  spline S868 degree 3 poles (119.1379, -90.4042) (119.0536, -90.4609) (118.9814, -90.538) (118.9302, -90.6286) knots 0 0 0 0 1 1 1 1
  spline S869 degree 3 poles (118.9302, -90.6286) (118.8791, -90.7191) (118.849, -90.823) (118.8451, -90.9282) knots 0 0 0 0 1 1 1 1
  spline S870 degree 3 poles (118.8451, -90.9282) (118.8408, -91.0314) (118.8626, -91.1352) (118.9052, -91.2281) knots 0 0 0 0 1 1 1 1
  spline S871 degree 3 poles (118.9052, -91.2281) (118.9478, -91.3211) (119.0114, -91.403) (119.0885, -91.4668) knots 0 0 0 0 1 1 1 1
  spline S872 degree 3 poles (119.0885, -91.4668) (119.2426, -91.5944) (119.4489, -91.6453) (119.6429, -91.6153) knots 0 0 0 0 1 1 1 1
  spline S873 degree 3 poles (119.6429, -91.6153) (119.7892, -91.5927) (119.9302, -91.5248) (120.0366, -91.4168) knots 0 0 0 0 1 1 1 1
  spline S874 degree 3 poles (120.0366, -91.4168) (120.1431, -91.3087) (120.2134, -91.1599) (120.2231, -91.0046) knots 0 0 0 0 1 1 1 1
  spline S875 degree 3 poles (120.2231, -91.0046) (120.2327, -90.8478) (120.1808, -90.6891) (120.087, -90.5668) knots 0 0 0 0 1 1 1 1
  spline S876 degree 3 poles (120.087, -90.5668) (119.9932, -90.4445) (119.8596, -90.3583) (119.7154, -90.3175) knots 0 0 0 0 1 1 1 1
  spline S877 degree 3 poles (49.0189, -107.8726) (49.8748, -106.8886) (48.7959, -104.7167) (49.8274, -104.7075) knots 0 0 0 0 1 1 1 1
  spline S878 degree 3 poles (49.8274, -104.7075) (54.9018, -104.6626) (66.1684, -104.2435) (67.995, -104.8049) knots 0 0 0 0 1 1 1 1
  spline S879 degree 3 poles (67.995, -104.8049) (70.5733, -105.5972) (72.4007, -106.5302) (74.9862, -108.8463) knots 0 0 0 0 1 1 1 1
  spline S880 degree 3 poles (74.9862, -108.8463) (76.1496, -109.8885) (76.4991, -112.2407) (76.0801, -113.7642) knots 0 0 0 0 1 1 1 1
  spline S881 degree 3 poles (76.0801, -113.7642) (75.5252, -115.7817) (73.5254, -117.3204) (72.1802, -117.4648) knots 0 0 0 0 1 1 1 1
  spline S882 degree 3 poles (72.1802, -117.4648) (69.4484, -117.7579) (63.8433, -117.4165) (59.7197, -117.9517) knots 0 0 0 0 1 1 1 1
  spline S883 degree 3 poles (59.7197, -117.9517) (58.9794, -118.0477) (58.2706, -118.3297) (57.532, -118.4386) knots 0 0 0 0 1 1 1 1
  spline S884 degree 3 poles (57.532, -118.4386) (56.6667, -118.5664) (55.753, -118.3739) (54.9162, -118.6332) knots 0 0 0 0 1 1 1 1
  spline S885 degree 3 poles (54.9162, -118.6332) (53.4689, -119.0816) (52.087, -121.0598) (50.9688, -120.9217) knots 0 0 0 0 1 1 1 1
  spline S886 degree 3 poles (50.9688, -120.9217) (49.3438, -120.7209) (44.1004, -112.9737) (44.263, -111.2807) knots 0 0 0 0 1 1 1 1
  spline S887 degree 3 poles (44.263, -111.2807) (44.5443, -109.8269) (48.3069, -108.6912) (49.0189, -107.8726) knots 0 0 0 0 1 1 1 1
  spline S888 degree 3 poles (70.801, -108.7004) (69.2549, -108.7684) (67.4814, -110.2327) (67.6146, -112.1575) knots 0 0 0 0 1 1 1 1
  spline S889 degree 3 poles (67.6146, -112.1575) (67.7325, -113.8636) (69.2812, -115.8931) (71.229, -115.712) knots 0 0 0 0 1 1 1 1
  spline S890 degree 3 poles (71.229, -115.712) (73.1541, -115.5331) (74.4104, -113.8341) (74.3204, -111.914) knots 0 0 0 0 1 1 1 1
  spline S891 degree 3 poles (74.3204, -111.914) (74.2195, -109.7647) (72.3715, -108.6311) (70.801, -108.7004) knots 0 0 0 0 1 1 1 1
  spline S892 degree 3 poles (65.2991, -114.9001) (65.0056, -114.9083) (64.6689, -115.1783) (64.6942, -115.5279) knots 0 0 0 0 1 1 1 1
  spline S893 degree 3 poles (64.6942, -115.5279) (64.7168, -115.8375) (65.0106, -116.2063) (65.3803, -116.1734) knots 0 0 0 0 1 1 1 1
  spline S894 degree 3 poles (65.3803, -116.1734) (65.7458, -116.1405) (65.9843, -115.8325) (65.9672, -115.4837) knots 0 0 0 0 1 1 1 1
  spline S895 degree 3 poles (65.9672, -115.4837) (65.9483, -115.0933) (65.5972, -114.8875) (65.2991, -114.9001) knots 0 0 0 0 1 1 1 1
  spline S896 degree 3 poles (67.3442, -105.9407) (67.0506, -105.949) (66.714, -106.219) (66.7393, -106.5686) knots 0 0 0 0 1 1 1 1
  spline S897 degree 3 poles (66.7393, -106.5686) (66.7618, -106.8782) (67.0557, -107.247) (67.4254, -107.2141) knots 0 0 0 0 1 1 1 1
  spline S898 degree 3 poles (67.4254, -107.2141) (67.7909, -107.1812) (68.0294, -106.8732) (68.0122, -106.5244) knots 0 0 0 0 1 1 1 1
  spline S899 degree 3 poles (68.0122, -106.5244) (67.9933, -106.134) (67.6423, -105.9282) (67.3442, -105.9407) knots 0 0 0 0 1 1 1 1
  line L255 (48.7098, -112.5227) -> (51.064, -111.208)
  line L256 (51.064, -111.208) -> (53.323, -114.7624)
  line L257 (53.323, -114.7624) -> (50.9213, -116.3206)
  line L258 (50.9213, -116.3206) -> (48.7098, -112.5227)
  spline S900 degree 3 poles (16.5894, -70.3403) (17.054, -70.3925) (18.3396, -72.3718) (18.7525, -72.3755) knots 0 0 0 0 1 1 1 1
  spline S901 degree 3 poles (18.7525, -72.3755) (19.109, -72.3788) (19.2494, -72.0129) (19.49, -72.0532) knots 0 0 0 0 1 1 1 1
  spline S902 degree 2 poles (19.49, -72.0532) (21.0863, -73.8966) (20.5855, -74.6488) knots 0 0 0 1 1 1
  spline S903 degree 3 poles (20.5855, -74.6488) (11.5818, -88.1751) (13.0317, -100.427) (14.1093, -117.5916) knots 0 0 0 0 1 1 1 1
  spline S904 degree 3 poles (14.1093, -117.5916) (14.3212, -120.9663) (14.235, -124.438) (13.6843, -127.7882) knots 0 0 0 0 1 1 1 1
  spline S905 degree 3 poles (13.6843, -127.7882) (11.3884, -141.7539) (8.68, -152.0088) (17.376, -168.2552) knots 0 0 0 0 1 1 1 1
  spline S906 degree 3 poles (17.376, -168.2552) (17.6739, -168.8117) (16.3953, -169.6486) (16.0313, -169.7944) knots 0 0 0 0 1 1 1 1
  spline S907 degree 3 poles (16.0313, -169.7944) (15.668, -169.9394) (15.1374, -169.563) (14.7376, -169.7577) knots 0 0 0 0 1 1 1 1
  spline S908 degree 3 poles (14.7376, -169.7577) (14.3649, -169.941) (13.7441, -171.0829) (13.2909, -171.2001) knots 0 0 0 0 1 1 1 1
  spline S909 degree 3 poles (13.2909, -171.2001) (12.8541, -171.313) (10.8754, -169.3092) (10.8851, -168.8867) knots 0 0 0 0 1 1 1 1
  spline S910 degree 3 poles (10.8851, -168.8867) (10.8924, -168.5615) (11.7748, -167.4545) (11.9848, -166.5976) knots 0 0 0 0 1 1 1 1
  spline S911 degree 3 poles (11.9848, -166.5976) (11.267, -165.7455) (11.209, -165.7087) (10.704, -165.1846) knots 0 0 0 0 1 1 1 1
  spline S912 degree 3 poles (10.704, -165.1846) (9.5235, -165.5501) (9.0786, -166.5331) (8.5043, -166.5053) knots 0 0 0 0 1 1 1 1
  spline S913 degree 3 poles (8.5043, -166.5053) (7.9704, -166.4809) (6.9962, -165.7656) (6.9001, -165.4127) knots 0 0 0 0 1 1 1 1
  spline S914 degree 3 poles (6.9001, -165.4127) (3.7455, -145.2091) (8.8533, -139.256) (9.7579, -126.1664) knots 0 0 0 0 1 1 1 1
  spline S915 degree 3 poles (9.7579, -126.1664) (10.6567, -113.1612) (8.9759, -109.1372) (8.2796, -97.2077) knots 0 0 0 0 1 1 1 1
  spline S916 degree 3 poles (8.2796, -97.2077) (7.8944, -90.6085) (7.0026, -89.8499) (10.7981, -74.8395) knots 0 0 0 0 1 1 1 1
  spline S917 degree 3 poles (10.7981, -74.8395) (11.3395, -74.2965) (12.6531, -76.325) (13.5765, -76.8342) knots 0 0 0 0 1 1 1 1
  spline S918 degree 3 poles (13.5765, -76.8342) (14.8905, -76.0421) (14.8981, -75.9994) (15.7966, -75.1331) knots 0 0 0 0 1 1 1 1
  spline S919 degree 3 poles (15.7966, -75.1331) (15.1026, -74.2018) (14.3323, -72.9608) (14.3082, -72.6124) knots 0 0 0 0 1 1 1 1
  spline S920 degree 3 poles (14.3082, -72.6124) (14.2825, -72.2424) (16.1779, -70.2922) (16.5894, -70.3386) knots 0 0 0 0 1 1 1 1
  line L259 (16.5894, -70.3386) -> (16.5894, -70.3403)
  spline S921 degree 3 poles (82.8193, -15.7332) (83.2099, -15.1441) (83.7092, -14.6273) (84.2844, -14.2164) knots 0 0 0 0 1 1 1 1
  spline S922 degree 3 poles (84.2844, -14.2164) (85.4885, -13.3564) (86.9749, -12.9875) (88.442, -12.7947) knots 0 0 0 0 1 1 1 1
  spline S923 degree 3 poles (88.442, -12.7947) (90.8719, -12.4752) (93.3559, -12.5925) (95.7514, -13.1104) knots 0 0 0 0 1 1 1 1
  spline S924 degree 3 poles (95.7514, -13.1104) (99.2028, -13.8565) (102.4668, -15.4383) (105.2112, -17.6602) knots 0 0 0 0 1 1 1 1
  spline S925 degree 3 poles (105.2112, -17.6602) (107.3575, -19.3979) (109.1884, -21.5238) (110.5886, -23.9039) knots 0 0 0 0 1 1 1 1
  line L260 (110.5886, -23.9039) -> (110.5322, -35.0778)
  line L261 (110.5322, -35.0778) -> (113.2596, -35.1226)
  line L262 (113.2596, -35.1226) -> (113.1916, -38.0651)
  line L263 (113.1916, -38.0651) -> (110.3165, -38.1886)
  line L264 (110.3165, -38.1886) -> (110.1315, -49.4205)
  spline S926 degree 3 poles (110.1315, -49.4205) (108.9186, -51.2018) (107.4797, -52.8293) (105.8603, -54.2514) knots 0 0 0 0 1 1 1 1
  spline S927 degree 3 poles (105.8603, -54.2514) (103.7443, -56.1097) (101.294, -57.6269) (98.598, -58.4409) knots 0 0 0 0 1 1 1 1
  spline S928 degree 3 poles (98.598, -58.4409) (96.6259, -59.0363) (94.5582, -59.2477) (92.5006, -59.3472) knots 0 0 0 0 1 1 1 1
  spline S929 degree 3 poles (92.5006, -59.3472) (89.7869, -59.4783) (86.941, -59.3896) (84.5518, -58.096) knots 0 0 0 0 1 1 1 1
  spline S930 degree 3 poles (84.5518, -58.096) (83.47, -57.5104) (82.5166, -56.6891) (81.7773, -55.706) knots 0 0 0 0 1 1 1 1
  line L265 (81.7773, -55.706) -> (92.3621, -55.7427)
  line L266 (92.3621, -55.7427) -> (93.0192, -43.1829)
  line L267 (93.0192, -43.1829) -> (97.5253, -43.0936)
  line L268 (97.5253, -43.0936) -> (97.8305, -28.991)
  line L269 (97.8305, -28.991) -> (93.1319, -28.9111)
  line L270 (93.1319, -28.9111) -> (92.9395, -15.7202)
  line L271 (92.9395, -15.7202) -> (82.8193, -15.7332)
  spline S931 degree 3 poles (22.8987, -126.766) (21.6974, -127.1032) (20.4249, -127.1598) (19.2006, -126.9306) knots 0 0 0 0 1 1 1 1
  spline S932 degree 3 poles (19.2006, -126.9306) (18.7885, -126.8534) (18.3796, -126.7434) (17.9983, -126.5627) knots 0 0 0 0 1 1 1 1
  spline S933 degree 3 poles (17.9983, -126.5627) (17.6169, -126.3821) (17.2628, -126.128) (16.9942, -125.7922) knots 0 0 0 0 1 1 1 1
  spline S934 degree 3 poles (16.9942, -125.7922) (16.6282, -125.3346) (16.4379, -124.748) (16.3436, -124.1596) knots 0 0 0 0 1 1 1 1
  spline S935 degree 3 poles (16.3436, -124.1596) (16.2493, -123.5712) (16.2435, -122.9718) (16.203, -122.3767) knots 0 0 0 0 1 1 1 1
  spline S936 degree 3 poles (16.203, -122.3767) (16.1646, -121.8119) (16.0946, -121.2479) (16.1054, -120.6818) knots 0 0 0 0 1 1 1 1
  spline S937 degree 3 poles (16.1054, -120.6818) (16.1162, -120.1157) (16.2128, -119.5386) (16.4847, -119.0489) knots 0 0 0 0 1 1 1 1
  spline S938 degree 3 poles (16.4847, -119.0489) (16.6872, -118.6844) (16.984, -118.3779) (17.3351, -118.1709) knots 0 0 0 0 1 1 1 1
  spline S939 degree 3 poles (17.3351, -118.1709) (17.6862, -117.9639) (18.0906, -117.857) (18.4936, -117.8645) knots 0 0 0 0 1 1 1 1
  line L272 (18.4936, -117.8645) -> (26.0033, -117.606)
  spline S940 degree 3 poles (26.0033, -117.606) (26.3003, -117.596) (26.5981, -117.587) (26.892, -117.5418) knots 0 0 0 0 1 1 1 1
  spline S941 degree 3 poles (26.892, -117.5418) (27.1859, -117.4964) (27.4787, -117.412) (27.7321, -117.2498) knots 0 0 0 0 1 1 1 1
  spline S942 degree 3 poles (27.7321, -117.2498) (28.0816, -117.0262) (28.3415, -116.6542) (28.4391, -116.2379) knots 0 0 0 0 1 1 1 1
  line L273 (28.4391, -116.2379) -> (28.6882, -113.9673)
  spline S943 degree 3 poles (28.6882, -113.9673) (30.1271, -113.7155) (31.6192, -113.8023) (33.0226, -114.2192) knots 0 0 0 0 1 1 1 1
  spline S944 degree 3 poles (33.0226, -114.2192) (35.0943, -114.8347) (36.9826, -116.205) (38.1219, -118.1164) knots 0 0 0 0 1 1 1 1
  spline S945 degree 3 poles (38.1219, -118.1164) (38.8813, -119.3906) (39.2987, -120.8852) (39.3143, -122.3866) knots 0 0 0 0 1 1 1 1
  line L274 (39.3143, -122.3866) -> (39.7495, -129.4487)
  spline S946 degree 3 poles (39.7495, -129.4487) (39.8968, -130.1298) (40.2886, -130.75) (40.8299, -131.1589) knots 0 0 0 0 1 1 1 1
  spline S947 degree 3 poles (40.8299, -131.1589) (41.116, -131.3751) (41.4431, -131.5314) (41.7865, -131.6171) knots 0 0 0 0 1 1 1 1
  spline S948 degree 3 poles (41.7865, -131.6171) (42.1298, -131.7028) (42.4857, -131.7135) (42.8387, -131.7151) knots 0 0 0 0 1 1 1 1
  line L275 (42.8387, -131.7151) -> (57.1926, -131.777)
  spline S949 degree 3 poles (57.1926, -131.777) (58.1552, -131.747) (59.1184, -132.2499) (59.674, -133.0725) knots 0 0 0 0 1 1 1 1
  spline S950 degree 3 poles (59.674, -133.0725) (60.0615, -133.6464) (60.2503, -134.3477) (60.3036, -135.0481) knots 0 0 0 0 1 1 1 1
  spline S951 degree 3 poles (60.3036, -135.0481) (60.3354, -135.4652) (60.3216, -135.8859) (60.3726, -136.3009) knots 0 0 0 0 1 1 1 1
  spline S952 degree 3 poles (60.3726, -136.3009) (60.4236, -136.7159) (60.5469, -137.1359) (60.8136, -137.4478) knots 0 0 0 0 1 1 1 1
  spline S953 degree 3 poles (60.8136, -137.4478) (61.0579, -137.7337) (61.4048, -137.9063) (61.7612, -137.9965) knots 0 0 0 0 1 1 1 1
  spline S954 degree 3 poles (61.7612, -137.9965) (62.1175, -138.0866) (62.4869, -138.1008) (62.8533, -138.1144) knots 0 0 0 0 1 1 1 1
  spline S955 degree 3 poles (62.8533, -138.1144) (74.0678, -138.5311) (85.2874, -138.7978) (96.5084, -138.9143) knots 0 0 0 0 1 1 1 1
  spline S956 degree 3 poles (96.5084, -138.9143) (96.9637, -138.8364) (97.4021, -138.653) (97.7832, -138.3811) knots 0 0 0 0 1 1 1 1
  spline S957 degree 3 poles (97.7832, -138.3811) (98.1102, -138.1477) (98.3948, -137.8497) (98.6176, -137.5075) knots 0 0 0 0 1 1 1 1
  line L276 (98.6176, -137.5075) -> (99.2242, -134.4096)
  spline S958 degree 3 poles (99.2242, -134.4096) (99.3482, -134.0207) (99.5663, -133.665) (99.8525, -133.3849) knots 0 0 0 0 1 1 1 1
  spline S959 degree 3 poles (99.8525, -133.3849) (100.3085, -132.9386) (100.9386, -132.693) (101.5626, -132.7183) knots 0 0 0 0 1 1 1 1
  line L277 (101.5626, -132.7183) -> (106.4661, -132.6483)
  spline S960 degree 3 poles (106.4661, -132.6483) (107.1986, -132.7124) (107.9527, -132.4204) (108.4685, -131.8727) knots 0 0 0 0 1 1 1 1
  spline S961 degree 3 poles (108.4685, -131.8727) (108.8495, -131.468) (109.0964, -130.9418) (109.2479, -130.3964) knots 0 0 0 0 1 1 1 1
  spline S962 degree 3 poles (109.2479, -130.3964) (109.3994, -129.851) (109.4602, -129.2833) (109.5192, -128.7187) knots 0 0 0 0 1 1 1 1
  line L278 (109.5192, -128.7187) -> (110.1876, -122.3261)
  spline S963 degree 3 poles (110.1876, -122.3261) (110.4294, -121.0308) (110.9624, -119.796) (111.7313, -118.7495) knots 0 0 0 0 1 1 1 1
  spline S964 degree 3 poles (111.7313, -118.7495) (113.3218, -116.5848) (115.9282, -115.3033) (118.5386, -115.3152) knots 0 0 0 0 1 1 1 1
  spline S965 degree 3 poles (118.5386, -115.3152) (119.3044, -115.3185) (120.0697, -115.4266) (120.8091, -115.6352) knots 0 0 0 0 1 1 1 1
  line L279 (120.8091, -115.6352) -> (121.019, -117.9555)
  spline S966 degree 3 poles (121.019, -117.9555) (121.0502, -118.3644) (121.2168, -118.7607) (121.4839, -119.0611) knots 0 0 0 0 1 1 1 1
  spline S967 degree 3 poles (121.4839, -119.0611) (121.7959, -119.4121) (122.2306, -119.6237) (122.6773, -119.731) knots 0 0 0 0 1 1 1 1
  spline S968 degree 3 poles (122.6773, -119.731) (123.1239, -119.8384) (123.5862, -119.8488) (124.0445, -119.8496) knots 0 0 0 0 1 1 1 1
  spline S969 degree 3 poles (124.0445, -119.8496) (125.9149, -119.8529) (127.7884, -119.7039) (129.6536, -119.8496) knots 0 0 0 0 1 1 1 1
  spline S970 degree 3 poles (129.6536, -119.8496) (129.9474, -119.8724) (130.2417, -119.903) (130.5281, -119.9749) knots 0 0 0 0 1 1 1 1
  spline S971 degree 3 poles (130.5281, -119.9749) (130.8145, -120.0469) (131.094, -120.162) (131.3328, -120.3424) knots 0 0 0 0 1 1 1 1
  spline S972 degree 3 poles (131.3328, -120.3424) (131.6699, -120.5971) (131.9123, -120.9732) (132.0614, -121.3793) knots 0 0 0 0 1 1 1 1
  spline S973 degree 3 poles (132.0614, -121.3793) (132.2105, -121.7853) (132.2713, -122.2216) (132.2934, -122.656) knots 0 0 0 0 1 1 1 1
  spline S974 degree 3 poles (132.2934, -122.656) (132.3358, -123.489) (132.2397, -124.322) (132.2032, -125.1553) knots 0 0 0 0 1 1 1 1
  spline S975 degree 3 poles (132.2032, -125.1553) (132.1749, -125.8024) (132.1821, -126.4552) (132.0625, -127.0907) knots 0 0 0 0 1 1 1 1
  spline S976 degree 3 poles (132.0625, -127.0907) (131.9429, -127.7263) (131.6809, -128.3568) (131.2066, -128.7732) knots 0 0 0 0 1 1 1 1
  spline S977 degree 3 poles (131.2066, -128.7732) (130.7702, -129.1564) (130.1918, -129.3248) (129.623, -129.3612) knots 0 0 0 0 1 1 1 1
  spline S978 degree 3 poles (129.623, -129.3612) (129.0543, -129.3977) (128.4857, -129.3131) (127.9197, -129.2446) knots 0 0 0 0 1 1 1 1
  spline S979 degree 3 poles (127.9197, -129.2446) (127.5161, -129.1957) (127.1096, -129.1546) (126.7171, -129.045) knots 0 0 0 0 1 1 1 1
  spline S980 degree 3 poles (126.7171, -129.045) (126.6159, -129.0168) (126.5125, -128.9821) (126.4341, -128.9095) knots 0 0 0 0 1 1 1 1
  spline S981 degree 3 poles (126.4341, -128.9095) (126.3589, -128.8398) (126.3126, -128.7374) (126.3088, -128.6325) knots 0 0 0 0 1 1 1 1
  line L280 (126.3088, -128.6325) -> (126.1736, -126.2004)
  spline S982 degree 3 poles (126.1736, -126.2004) (126.163, -126.0123) (126.0628, -125.8319) (125.9112, -125.7301) knots 0 0 0 0 1 1 1 1
  spline S983 degree 3 poles (125.9112, -125.7301) (125.8074, -125.6604) (125.6817, -125.6272) (125.5587, -125.6369) knots 0 0 0 0 1 1 1 1
  line L281 (125.5587, -125.6369) -> (122.0962, -125.6752)
  spline S984 degree 3 poles (122.0962, -125.6752) (121.958, -125.6797) (121.823, -125.7517) (121.7394, -125.8669) knots 0 0 0 0 1 1 1 1
  spline S985 degree 3 poles (121.7394, -125.8669) (121.6998, -125.9214) (121.6717, -125.9847) (121.6551, -126.0509) knots 0 0 0 0 1 1 1 1
  spline S986 degree 3 poles (121.6551, -126.0509) (121.6385, -126.1171) (121.634, -126.1859) (121.6306, -126.2543) knots 0 0 0 0 1 1 1 1
  line L282 (121.6306, -126.2543) -> (121.0299, -138.5049)
  spline S987 degree 3 poles (121.0299, -138.5049) (121.0943, -139.6441) (120.7108, -140.8039) (119.9875, -141.6582) knots 0 0 0 0 1 1 1 1
  spline S988 degree 3 poles (119.9875, -141.6582) (119.2511, -142.5279) (118.1713, -143.0694) (117.0618, -143.1254) knots 0 0 0 0 1 1 1 1
  line L283 (117.0618, -143.1254) -> (107.9216, -144.0748)
  spline S989 degree 3 poles (107.9216, -144.0748) (107.8168, -144.0671) (107.7097, -144.1047) (107.6299, -144.1762) knots 0 0 0 0 1 1 1 1
  spline S990 degree 3 poles (107.6299, -144.1762) (107.5737, -144.2266) (107.5337, -144.2934) (107.4975, -144.361) knots 0 0 0 0 1 1 1 1
  line L284 (107.4975, -144.361) -> (107.3443, -144.6471)
  line L285 (107.3443, -144.6471) -> (45.253, -143.7839)
  spline S991 degree 3 poles (45.253, -143.7839) (43.5865, -143.7607) (41.916, -143.5735) (40.3199, -143.0716) knots 0 0 0 0 1 1 1 1
  spline S992 degree 3 poles (40.3199, -143.0716) (39.2963, -142.7497) (38.2971, -142.3426) (37.3351, -141.8555) knots 0 0 0 0 1 1 1 1
  line L286 (37.3351, -141.8555) -> (32.1302, -141.7141)